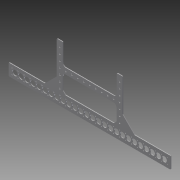
# Autodesk Inventor part: Strength Plate (0.125 Steel)
Saved by Autodesk Inventor 2014 (Build 180170000, 170)
## iProperties
Created: 2014-02-09
Part Number: Strength Plate (0.125 Steel)
Material: Steel
Document SubType Name: Modeling
Designer: Andrew Toennies
Mass: 1038.79 g
Surface Area: 1009.7 cm^2
Volume: 132.33 cm^3
Density: 7.85 g/cm^3
Appearance: Steel
Author: Andrew Toennies
Autodesk Inventor part; units mm, degrees
ref_plane "YZ Plane" through (0, 0, 0) normal (1, 0, 0) x (0, 1, 0)
ref_plane "XZ Plane" through (0, 0, 0) normal (0, 1, 0) x (-1, 0, 0)
ref_plane "XY Plane" through (0, 0, 0) normal (0, 0, 1) x (1, 0, 0)
sketch "Sketch1" plane through (0, 0, 0) normal (0, 0, 1) x (1, 0, 0)
  line L0 (3.175, 0) -> (685.8, 0)
  line L1 (688.975, 3.175) -> (688.975, 47.625)
  line L2 (0, 47.625) -> (0, 3.175)
  line L3 (204.7875, 102.9151) -> (204.7875, 238.125)
  line L4 (207.9625, 241.3) -> (227.0125, 241.3)
  line L5 (461.9625, 241.3) -> (481.0125, 241.3)
  line L6 (484.1875, 238.125) -> (484.1875, 102.9151)
  line L7 (203.8576, 100.6701) -> (154.9174, 51.7299)
  line L8 (231.1174, 61.2549) -> (240.6424, 51.7299)
  line L9 (457.8576, 61.2549) -> (448.3326, 51.7299)
  line L10 (485.1174, 100.6701) -> (534.0576, 51.7299)
  line L11 (152.6724, 50.8) -> (3.175, 50.8)
  line L12 (685.8, 50.8) -> (536.3026, 50.8)
  line L13 (446.0875, 50.8) -> (242.8875, 50.8)
  arc A0 (207.9625, 241.3) -> (204.7875, 238.125) centre (207.9625, 238.125) ccw
  arc A1 (230.1875, 238.125) -> (227.0125, 241.3) centre (227.0125, 238.125) ccw
  arc A2 (203.8576, 100.6701) -> (204.7875, 102.9151) centre (201.6125, 102.9151) ccw
  arc A3 (230.1875, 63.5) -> (231.1174, 61.2549) centre (233.3625, 63.5) ccw
  arc A4 (240.6424, 51.7299) -> (242.8875, 50.8) centre (242.8875, 53.975) ccw
  arc A5 (446.0875, 50.8) -> (448.3326, 51.7299) centre (446.0875, 53.975) ccw
  arc A6 (457.8576, 61.2549) -> (458.7875, 63.5) centre (455.6125, 63.5) ccw
  arc A7 (461.9625, 241.3) -> (458.7875, 238.125) centre (461.9625, 238.125) ccw
  arc A8 (484.1875, 238.125) -> (481.0125, 241.3) centre (481.0125, 238.125) ccw
  arc A9 (484.1875, 102.9151) -> (485.1174, 100.6701) centre (487.3625, 102.9151) ccw
  arc A10 (3.175, 50.8) -> (0, 47.625) centre (3.175, 47.625) ccw
  arc A11 (152.6724, 50.8) -> (154.9174, 51.7299) centre (152.6724, 53.975) ccw
  arc A12 (0, 3.175) -> (3.175, 0) centre (3.175, 3.175) ccw
  arc A13 (685.8, 0) -> (688.975, 3.175) centre (685.8, 3.175) ccw
  arc A14 (688.975, 47.625) -> (685.8, 50.8) centre (685.8, 47.625) ccw
  arc A15 (534.0576, 51.7299) -> (536.3026, 50.8) centre (536.3026, 53.975) ccw
  line L14 (242.8875, 152.4) -> (446.0875, 152.4)
  line L15 (242.8875, 127) -> (446.0875, 127)
  line L16 (458.7875, 63.5) -> (458.7875, 114.3)
  line L17 (458.7875, 165.1) -> (458.7875, 238.125)
  line L18 (230.1875, 238.125) -> (230.1875, 165.1)
  line L19 (230.1875, 114.3) -> (230.1875, 63.5)
  line L20 (228.8724, 63.5) -> (233.3625, 63.5) construction
  line L21 (455.6125, 63.5) -> (460.1026, 63.5) construction
  arc A16 (230.1875, 165.1) -> (242.8875, 152.4) centre (242.8875, 165.1) ccw
  arc A17 (242.8875, 127) -> (230.1875, 114.3) centre (242.8875, 114.3) ccw
  arc A18 (446.0875, 152.4) -> (458.7875, 165.1) centre (446.0875, 165.1) ccw
  arc A19 (458.7875, 114.3) -> (446.0875, 127) centre (446.0875, 114.3) ccw
  point P0 (0, 0)
  point P1 (688.975, 0)
  point P2 (688.975, 50.8)
  point P3 (153.9875, 50.8)
  point P4 (204.7875, 241.3)
  point P5 (231.5026, 241.3)
  point P6 (460.1026, 241.3)
  point P7 (484.1875, 241.3)
  point P8 (484.1875, 101.6)
  point P9 (204.7875, 101.6)
  point P10 (241.5724, 50.8)
  point P11 (534.9875, 50.8)
  point P12 (230.1875, 152.4)
  point P13 (458.7875, 152.4)
  point P14 (230.1875, 127)
  point P15 (458.7875, 127)
  dimension "d0" = 688.975
  dimension "d1" = 50.8
  dimension "d6" = 204.7875
  dimension "d7" = 204.7875
  dimension "d14" = 135
  dimension "d15" = 135
  dimension "d16" = 50.8
  dimension "d17" = 12.7
  dimension "d18" = 190.5
  dimension "d19" = 12.7
  dimension "d20" = 50.8
  dimension "d21" = 3.175
  dimension "d24" = 25.4
  dimension "d25" = 88.9
  dimension "d26" = 25.4
  dimension "d27" = 25.4
  dimension "d28" = 12.7
  constraints: 44 end point, 44 tangent, 40 point on circle, 32 point on line, 20 centre point, 19 perpendicular, 18 equal radius, 9 parallel, 3 collinear, 3 horizontal
  measures "d0" distance of point (0, 0) point (688.975, 0)
  measures "d1" distance of point (688.975, 0) point (688.975, 50.8)
  measures "d6" distance between parallel lines of L1 L6
  measures "d7" distance between parallel lines of L2 L3
  measures "d14" angle of L9 L13
  measures "d15" angle of L12 L10
  measures "d16" horizontal distance of point (204.788, 101.6) point (153.988, 50.8)
  measures "d17" horizontal distance of point (241.572, 50.8) L20.start
  measures "d18" distance between parallel lines of L13 L4
  measures "d19" distance from line of L13 L21.end
  measures "d20" horizontal distance of point (534.987, 50.8) point (484.188, 101.6)
  measures "d21" radius of A0
  measures "d24" distance between parallel lines of L14 L15
  measures "d25" distance between parallel lines of L4 L14
  measures "d26" distance between parallel lines of L17 L6
  measures "d27" distance between parallel lines of L3 L18
  measures "d28" radius of A16
extrude "Extrusion1" add sketch "Sketch1" along normal blind 3.175
sketch "Sketch2" plane through (0, 0, 3.175) normal (0, 0, 1) x (1, 0, 0)
  line L0 (242.8875, 127) -> (446.0875, 127) projected
  line L1 (204.7875, 238.125) -> (204.7875, 102.9151) projected
  line L2 (688.975, 3.175) -> (688.975, 47.625) projected
  line L3 (685.8, 50.8) -> (536.3026, 50.8) projected
  line L4 (446.0875, 152.4) -> (242.8875, 152.4) projected
  line L5 (230.1875, 165.1) -> (230.1875, 238.125) projected
  line L6 (227.0125, 241.3) -> (207.9625, 241.3) projected
  circle A0 centre (217.4875, 215.9) radius 3.3782
  circle A1 centre (217.4875, 190.5) radius 3.3782
  circle A2 centre (217.4875, 165.1) radius 3.3782
  circle A3 centre (217.4875, 139.7) radius 3.3782
  circle A4 centre (217.4875, 114.3) radius 3.3782
  circle A5 centre (217.4875, 88.9) radius 3.3782
  circle A6 centre (217.4875, 63.5) radius 3.3782
  circle A7 centre (242.8875, 139.7) radius 3.3782
  circle A8 centre (268.2875, 139.7) radius 3.3782
  circle A9 centre (293.6875, 139.7) radius 3.3782
  circle A10 centre (319.0875, 139.7) radius 3.3782
  circle A11 centre (344.4875, 139.7) radius 3.3782
  circle A12 centre (369.8875, 139.7) radius 3.3782
  circle A13 centre (395.2875, 139.7) radius 3.3782
  circle A14 centre (420.6875, 139.7) radius 3.3782
  circle A15 centre (446.0875, 139.7) radius 3.3782
  circle A16 centre (471.4875, 139.7) radius 3.3782
  line L7 (344.4875, 127) -> (344.4875, 70.4166) construction
  circle A17 centre (471.4875, 215.9) radius 3.3782
  circle A18 centre (471.4875, 190.5) radius 3.3782
  circle A19 centre (471.4875, 165.1) radius 3.3782
  circle A20 centre (471.4875, 114.3) radius 3.3782
  circle A21 centre (471.4875, 88.9) radius 3.3782
  circle A22 centre (471.4875, 63.5) radius 3.3782
  circle A23 centre (674.6875, 38.1) radius 2.0701
  circle A24 centre (674.6875, 12.7) radius 2.0701
  circle A25 centre (649.2875, 38.1) radius 2.0701
  circle A26 centre (649.2875, 12.7) radius 2.0701
  circle A27 centre (623.8875, 38.1) radius 2.0701
  circle A28 centre (623.8875, 12.7) radius 2.0701
  circle A29 centre (598.4875, 38.1) radius 2.0701
  circle A30 centre (598.4875, 12.7) radius 2.0701
  circle A31 centre (573.0875, 38.1) radius 2.0701
  circle A32 centre (573.0875, 12.7) radius 2.0701
  circle A33 centre (547.6875, 38.1) radius 2.0701
  circle A34 centre (547.6875, 12.7) radius 2.0701
  circle A35 centre (522.2875, 38.1) radius 2.0701
  circle A36 centre (522.2875, 12.7) radius 2.0701
  circle A37 centre (496.8875, 38.1) radius 2.0701
  circle A38 centre (496.8875, 12.7) radius 2.0701
  circle A39 centre (471.4875, 38.1) radius 2.0701
  circle A40 centre (471.4875, 12.7) radius 2.0701
  circle A41 centre (446.0875, 38.1) radius 2.0701
  circle A42 centre (446.0875, 12.7) radius 2.0701
  circle A43 centre (420.6875, 38.1) radius 2.0701
  circle A44 centre (420.6875, 12.7) radius 2.0701
  circle A45 centre (395.2875, 38.1) radius 2.0701
  circle A46 centre (395.2875, 12.7) radius 2.0701
  circle A47 centre (369.8875, 38.1) radius 2.0701
  circle A48 centre (369.8875, 12.7) radius 2.0701
  circle A49 centre (344.4875, 38.1) radius 2.0701
  circle A50 centre (344.4875, 12.7) radius 2.0701
  circle A51 centre (319.0875, 38.1) radius 2.0701
  circle A52 centre (319.0875, 12.7) radius 2.0701
  circle A53 centre (293.6875, 38.1) radius 2.0701
  circle A54 centre (293.6875, 12.7) radius 2.0701
  circle A55 centre (268.2875, 38.1) radius 2.0701
  circle A56 centre (268.2875, 12.7) radius 2.0701
  circle A57 centre (242.8875, 38.1) radius 2.0701
  circle A58 centre (242.8875, 12.7) radius 2.0701
  circle A59 centre (217.4875, 38.1) radius 2.0701
  circle A60 centre (217.4875, 12.7) radius 2.0701
  circle A61 centre (192.0875, 38.1) radius 2.0701
  circle A62 centre (192.0875, 12.7) radius 2.0701
  circle A63 centre (166.6875, 38.1) radius 2.0701
  circle A64 centre (166.6875, 12.7) radius 2.0701
  circle A65 centre (141.2875, 38.1) radius 2.0701
  circle A66 centre (141.2875, 12.7) radius 2.0701
  circle A67 centre (115.8875, 38.1) radius 2.0701
  circle A68 centre (115.8875, 12.7) radius 2.0701
  circle A69 centre (90.4875, 38.1) radius 2.0701
  circle A70 centre (90.4875, 12.7) radius 2.0701
  circle A71 centre (65.0875, 38.1) radius 2.0701
  circle A72 centre (65.0875, 12.7) radius 2.0701
  circle A73 centre (39.6875, 38.1) radius 2.0701
  circle A74 centre (39.6875, 12.7) radius 2.0701
  circle A75 centre (14.2875, 38.1) radius 2.0701
  circle A76 centre (14.2875, 12.7) radius 2.0701
  line L8 (3.175, 0) -> (685.8, 0) projected
  circle A77 centre (661.9875, 25.4) radius 11.1125
  circle A78 centre (636.5875, 25.4) radius 11.1125
  circle A79 centre (611.1875, 25.4) radius 11.1125
  circle A80 centre (585.7875, 25.4) radius 11.1125
  circle A81 centre (560.3875, 25.4) radius 11.1125
  circle A82 centre (534.9875, 25.4) radius 11.1125
  circle A83 centre (509.5875, 25.4) radius 11.1125
  circle A84 centre (484.1875, 25.4) radius 11.1125
  circle A85 centre (458.7875, 25.4) radius 11.1125
  circle A86 centre (433.3875, 25.4) radius 11.1125
  circle A87 centre (407.9875, 25.4) radius 11.1125
  circle A88 centre (382.5875, 25.4) radius 11.1125
  circle A89 centre (357.1875, 25.4) radius 11.1125
  circle A90 centre (331.7875, 25.4) radius 11.1125
  circle A91 centre (306.3875, 25.4) radius 11.1125
  circle A92 centre (280.9875, 25.4) radius 11.1125
  circle A93 centre (255.5875, 25.4) radius 11.1125
  circle A94 centre (230.1875, 25.4) radius 11.1125
  circle A95 centre (204.7875, 25.4) radius 11.1125
  circle A96 centre (179.3875, 25.4) radius 11.1125
  circle A97 centre (153.9875, 25.4) radius 11.1125
  circle A98 centre (128.5875, 25.4) radius 11.1125
  circle A99 centre (103.1875, 25.4) radius 11.1125
  circle A100 centre (77.7875, 25.4) radius 11.1125
  circle A101 centre (52.3875, 25.4) radius 11.1125
  circle A102 centre (26.9875, 25.4) radius 11.1125
  point P0 (0, 0)
  dimension "d29" = 6.7564
  dimension "d30" = 12.7
  dimension "d31" = 25.4
  dimension "d34" = 25.4
  dimension "d41" = 25.4
  dimension "d46" = 4.1402
  dimension "d47" = 12.7
  dimension "d48" = 14.2875
  dimension "d51" = 25.4
  dimension "d54" = 25.4
  dimension "d59" = 22.225
  dimension "d60" = 26.9875
  dimension "d61" = 25.4
  dimension "d64" = 25.4
  constraints: 103 centre point, 6 symmetric about line, 3 horizontal, 2 end point, 2 vertical, 1 midpoint, 1 perpendicular, 194 other
  measures "d29" diameter of A0
  measures "d30" distance from line of L5 A0.centre
  measures "d31" distance from line of L6 A0.centre
  measures "d34" distance of A0.centre A1.centre
  measures "d41" distance of A3.centre A7.centre
  measures "d46" diameter of A23
  measures "d47" distance from line of L3 A23.centre
  measures "d48" distance from line of L2 A23.centre
  measures "d51" distance of A23.centre A24.centre
  measures "d54" distance of A23.centre A25.centre
  measures "d59" diameter of A77
  measures "d60" distance from line of L2 A77.centre
  measures "d61" distance from line of L8 A77.centre
  measures "d64" distance of A77.centre A78.centre
extrude "Extrusion2" cut sketch "Sketch2" against normal blind 25.4
body "Solid1"
